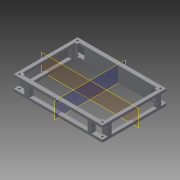
# Autodesk Inventor part: transillum_diffusor_partD2_v1
Saved by Autodesk Inventor 2015 (Build 190159000, 159)
## iProperties
Created: 2022-06-08
Part Number: transillum_diffusor_partD2_v1
Material: Genérico
Document SubType Name: Modeling
Designer: Zuloaga
Density: 1 g/cm^3
Appearance: Valor por defecto
Author: Zuloaga
Autodesk Inventor part; units mm, degrees
ref_plane "YZ Plane" through (0, 0, 0) normal (1, 0, 0) x (0, 1, 0)
ref_plane "XZ Plane" through (0, 0, 0) normal (0, 1, 0) x (-1, 0, 0)
ref_plane "XY Plane" through (0, 0, 0) normal (0, 0, 1) x (1, 0, 0)
sketch "Boceto1" plane through (0, 0, 0) normal (0, 0, 1) x (1, 0, 0)
  line L0 (0, 0) -> (177, 0)
  line L1 (177, 0) -> (177, 127.5)
  line L2 (177, 127.5) -> (0, 127.5)
  line L3 (0, 127.5) -> (0, 0)
  line L4 (0, 127.5) -> (11.5, 127.5)
  line L5 (11.5, 127.5) -> (11.5, 116)
  line L6 (11.5, 116) -> (0, 116)
  line L7 (0, 116) -> (0, 127.5)
  line L8 (177, 0) -> (165.5, 0)
  line L9 (165.5, 0) -> (165.5, 11.5)
  line L10 (165.5, 11.5) -> (177, 11.5)
  line L11 (177, 11.5) -> (177, 0)
  line L12 (11.5, 116) -> (165.5, 116)
  line L13 (165.5, 116) -> (165.5, 11.5)
  line L14 (165.5, 11.5) -> (11.5, 11.5)
  line L15 (11.5, 11.5) -> (11.5, 116)
  dimension "d0" = 177
  dimension "d1" = 127.5
  dimension "d2" = 11.5
  dimension "d3" = 11.5
  dimension "d4" = 11.5
  dimension "d5" = 11.5
  constraints: 32 end point, 8 parallel, 4 horizontal, 4 perpendicular
  measures "d0" distance of L2.end L1.end
  measures "d1" distance of L1.end L0.end
  measures "d2" distance of L5.end L6.end
  measures "d3" distance of L4.end L5.end
  measures "d4" distance of L9.end L10.end
  measures "d5" distance of L8.end L9.end
extrude "Extrusión1" add sketch "Boceto1" along normal blind 30 contours L3 L6 L15 L14 L9 L0 | L9 L10 L1 L0 | L3 L2 L5 L6 | L13 L12 L5 L2 L1 L10
sketch "Boceto2" plane through (0, 0, 30) normal (0, 0, 1) x (1, 0, 0)
  line L0 (11.5, 116) -> (6.5, 116)
  line L1 (6.5, 116) -> (6.5, 11.5)
  line L2 (6.5, 11.5) -> (11.5, 11.5)
  line L3 (11.5, 11.5) -> (11.5, 116)
  line L4 (165.5, 116) -> (170.5, 116)
  line L5 (170.5, 116) -> (170.5, 11.5)
  line L6 (170.5, 11.5) -> (165.5, 11.5)
  line L7 (165.5, 11.5) -> (165.5, 116)
  line L8 (11.5, 116) -> (165.5, 116)
  line L9 (165.5, 116) -> (165.5, 119.75)
  line L10 (165.5, 119.75) -> (11.5, 119.75)
  line L11 (11.5, 119.75) -> (11.5, 116)
  line L12 (11.5, 11.5) -> (165.5, 11.5)
  line L13 (165.5, 11.5) -> (165.5, 7.75)
  line L14 (165.5, 7.75) -> (11.5, 7.75)
  line L15 (11.5, 7.75) -> (11.5, 11.5)
  dimension "d30" = 5
  dimension "d31" = 5
  dimension "d32" = 104.5
  dimension "d33" = 3.75
  dimension "d34" = 3.75
  constraints: 32 end point, 8 parallel, 4 horizontal, 4 perpendicular, 1 point on line
  measures "d30" distance of L2.end L1.end
  measures "d31" distance of L5.end L6.end
  measures "d32" distance of L4.end L5.end
  measures "d33" distance of L9.end L8.end
  measures "d34" distance of L12.end L13.end
extrude "Extrusión2" cut sketch "Boceto2" against normal blind 30 contours L3 L2 L1 L0 | L11 L10 L9 L8 | L12 L13 L14 L15 | L4 L5 L6 L7
sketch "Boceto3" plane through (0, 0, 30) normal (0, 0, 1) x (1, 0, 0)
  line L0 (177, 0) -> (171.25, 0)
  line L1 (171.25, 0) -> (171.25, 5.75)
  line L2 (171.25, 5.75) -> (177, 5.75)
  line L3 (177, 5.75) -> (177, 0)
  line L4 (0, 0) -> (5.75, 0)
  line L5 (5.75, 0) -> (5.75, 5.75)
  line L6 (5.75, 5.75) -> (0, 5.75)
  line L7 (0, 5.75) -> (0, 0)
  line L8 (0, 127.5) -> (5.75, 127.5)
  line L9 (5.75, 127.5) -> (5.75, 121.75)
  line L10 (5.75, 121.75) -> (0, 121.75)
  line L11 (0, 121.75) -> (0, 127.5)
  line L12 (177, 127.5) -> (171.25, 127.5)
  line L13 (171.25, 127.5) -> (171.25, 121.75)
  line L14 (171.25, 121.75) -> (177, 121.75)
  line L15 (177, 121.75) -> (177, 127.5)
  circle A0 centre (5.75, 121.75) radius 2
  circle A1 centre (171.25, 121.75) radius 2
  circle A2 centre (171.25, 5.75) radius 2
  circle A3 centre (5.75, 5.75) radius 2
  dimension "d16" = 5.75
  dimension "d17" = 5.75
  dimension "d18" = 5.75
  dimension "d19" = 5.75
  dimension "d20" = 5.75
  dimension "d21" = 5.75
  dimension "d22" = 5.75
  dimension "d23" = 5.75
  dimension "d24" = 4
  dimension "d25" = 4
  dimension "d26" = 4
  dimension "d27" = 4
  constraints: 32 end point, 8 parallel, 4 centre point, 4 coincident, 4 horizontal, 4 perpendicular
  measures "d16" distance of L1.end L2.end
  measures "d17" distance of L0.end L1.end
  measures "d18" distance of L6.end L5.end
  measures "d19" distance of L5.end L4.end
  measures "d20" distance of L9.end L10.end
  measures "d21" distance of L8.end L9.end
  measures "d22" distance of L14.end L13.end
  measures "d23" distance of L13.end L12.end
  measures "d24" diameter of A0
  measures "d25" diameter of A1
  measures "d26" diameter of A2
  measures "d27" diameter of A3
extrude "Extrusión3" cut sketch "Boceto3" against normal blind 30 contours A2 L2 L1 | L1 L2 A2 | A3 L6 L5 | L5 L6 A3 | A0 L10 L9 | L9 L10 A0 | A1 L14 L13 | L13 L14 A1
sketch "Boceto4" plane through (0, 0, 0) normal (0, -1, 0) x (1, 0, 0)
  line L0 (0, 30) -> (21.5, 30)
  line L1 (21.5, 30) -> (21.5, 0)
  line L2 (21.5, 0) -> (0, 0)
  line L3 (0, 0) -> (0, 30)
  line L4 (0, 30) -> (177, 30) projected
  line L5 (177, 0) -> (155.5, 0)
  line L6 (155.5, 0) -> (155.5, 30)
  line L7 (155.5, 30) -> (177, 30)
  line L8 (177, 30) -> (177, 0)
  line L9 (0, 30) -> (21.5, 30)
  line L10 (21.5, 30) -> (21.5, 25)
  line L11 (21.5, 25) -> (0, 25)
  line L12 (0, 25) -> (0, 30)
  line L13 (0, 0) -> (21.5, 0)
  line L14 (21.5, 0) -> (21.5, 5)
  line L15 (21.5, 5) -> (0, 5)
  line L16 (0, 5) -> (0, 0)
  line L17 (0, 25) -> (21.5, 25)
  line L18 (21.5, 25) -> (21.5, 5)
  line L19 (21.5, 5) -> (0, 5)
  line L20 (0, 5) -> (0, 25)
  dimension "d35" = 21.5
  dimension "d36" = 21.5
  dimension "d37" = 5
  dimension "d38" = 5
  constraints: 40 end point, 10 parallel, 5 horizontal, 5 perpendicular, 3 point on line
  measures "d35" distance of L1.end L2.end
  measures "d36" distance of L6.end L7.end
  measures "d37" distance of L9.end L10.end
  measures "d38" distance of L14.end L13.end
extrude "Extrusión4" cut sketch "Boceto4" against normal blind 10.5 contours L11 L1 L15 L3
ref_plane "Plano de trabajo1" through (88.5, 0, 0) normal (-1, 0, 0) x (0, 0, 1)
ref_plane "Plano de trabajo2" through (11.5, 63.75, 30) normal (0, -1, 0) x (1, 0, 0)
mirror "Simetría1" about plane through (88.5, 0, 0) normal (-1, 0, 0) of "Extrusión4"
mirror "Simetría2" about plane through (11.5, 63.75, 30) normal (0, -1, 0) of "Extrusión4", "Simetría1"
sketch "Boceto5" plane through (0, 0, 0) normal (0, -1, 0) x (1, 0, 0)
  line L0 (21.5, 25) -> (155.5, 25)
  line L1 (155.5, 25) -> (155.5, 5)
  line L2 (155.5, 5) -> (21.5, 5)
  line L3 (21.5, 5) -> (21.5, 25)
  line L4 (21.5, 25) -> (31.5, 25)
  line L5 (31.5, 25) -> (31.5, 5)
  line L6 (31.5, 5) -> (21.5, 5)
  line L7 (21.5, 5) -> (21.5, 25)
  line L8 (155.5, 5) -> (147.5, 5)
  line L9 (147.5, 5) -> (147.5, 25)
  line L10 (147.5, 25) -> (155.5, 25)
  line L11 (155.5, 25) -> (155.5, 5)
  line L12 (31.5, 25) -> (147.5, 25)
  line L13 (147.5, 25) -> (147.5, 5)
  line L14 (147.5, 5) -> (31.5, 5)
  line L15 (31.5, 5) -> (31.5, 25)
  point P0 (0, 0)
  dimension "d41" = 10
  dimension "d42" = 8
  constraints: 32 end point, 8 parallel, 4 horizontal, 4 perpendicular, 2 point on line
  measures "d41" distance of L5.end L6.end
  measures "d42" distance of L9.end L10.end
extrude "Extrusión5" cut sketch "Boceto5" against normal blind 11.5 contours L0 L9 L2 L5
sketch "Boceto6" plane through (177, 0, 0) normal (1, 0, 0) x (0, 0, -1)
  line L0 (-25, 10.5) -> (-5, 10.5)
  line L1 (-5, 10.5) -> (-5, 18.5)
  line L2 (-5, 18.5) -> (-25, 18.5)
  line L3 (-25, 18.5) -> (-25, 10.5)
  line L4 (-25, 117) -> (-5, 117)
  line L5 (-5, 117) -> (-5, 109)
  line L6 (-5, 109) -> (-25, 109)
  line L7 (-25, 109) -> (-25, 117)
  line L8 (-25, 109) -> (-5, 109)
  line L9 (-5, 109) -> (-5, 18.5)
  line L10 (-5, 18.5) -> (-25, 18.5)
  line L11 (-25, 18.5) -> (-25, 109)
  point P0 (0, 0)
  dimension "d45" = 20
  dimension "d46" = 8
  dimension "d47" = 20
  dimension "d48" = 8
  constraints: 24 end point, 6 parallel, 3 horizontal, 3 perpendicular
  measures "d45" distance of L2.end L1.end
  measures "d46" distance of L1.end L0.end
  measures "d47" distance of L5.end L6.end
  measures "d48" distance of L4.end L5.end
extrude "Extrusión6" cut sketch "Boceto6" against normal blind 200 contours L11 L6 L9 L2
